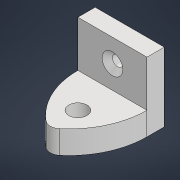
# Autodesk Inventor part: Winkel
Saved by Autodesk Inventor 2021 (Build 250183000, 183)
## iProperties
Created: 2023-10-25
Part Number: Winkel
Material: Generisch
Document SubType Name: Modeling
Designer: Tobias Sauter
Density: 1 g/cm^3
Appearance: Vorgabe
Author: Team 8
Autodesk Inventor part; units mm, degrees
ref_plane "YZ Plane" through (0, 0, 0) normal (1, 0, 0) x (0, 1, 0)
ref_plane "XZ Plane" through (0, 0, 0) normal (0, 1, 0) x (-1, 0, 0)
ref_plane "XY Plane" through (0, 0, 0) normal (0, 0, 1) x (1, 0, 0)
sketch "Skizze2" plane through (0, 0, 0) normal (0, 0, 1) x (1, 0, 0)
  line L0 (-36, 116.4167) -> (-56, 116.4167)
  line L1 (-56, 116.4167) -> (-56, 96.4167)
  line L2 (-56, 96.4167) -> (-36, 96.4167)
  line L3 (-36, 96.4167) -> (-36, 116.4167)
  circle A0 centre (-46, 109.75) radius 1.7 projected
  point P0 (0, 0)
  dimension "d0" = 20
  dimension "d1" = 10
  dimension "d2" = 20
  dimension "d3" = 6.6667
  constraints: 8 end point, 2 parallel, 1 horizontal, 1 perpendicular
  measures "d0" distance of L0.start L0.end
  measures "d1" distance from line of L3 A0.centre
  measures "d2" distance of L0.end L1.end
  measures "d3" distance from line of L0 A0.centre
extrude "Extrusion1" add sketch "Skizze2" along normal blind 5 contours L3 L2 L1 L0 | A0
sketch "Skizze4" plane through (-56, 96.4167, 0) normal (0, -1, 0) x (1, 0, 0)
  line L0 (0, 0) -> (20, 0) projected
  line L1 (20, 0) -> (20, 5) projected
  line L2 (0, 5) -> (20, 5) projected
  line L3 (0, 0) -> (0, 5) projected
  line L4 (0, 0) -> (0, 5) projected
  line L5 (20, 0) -> (20, 5) projected
  arc A0 (11.927, 22.2993) -> (8.073, 22.2993) centre (10, 20) ccw
  line L6 (10, 20) -> (10, 5) construction
  line L7 (0, 5) -> (20, 5) construction
  arc A1 (8.073, 22.2993) -> (0, 5) centre (22.5714, 5) ccw
  arc A2 (20, 5) -> (11.927, 22.2993) centre (-2.5714, 5) ccw
  circle A3 centre (10, 15) radius 2.65
  point P0 (56, 0)
  dimension "d6" = 6
  dimension "d7" = 15
  dimension "d8" = 23
  dimension "d11" = 5.3
  dimension "d20" = 10
  constraints: 6 point on circle, 4 centre point, 2 end point, 2 symmetric about line, 2 tangent, 1 midpoint, 1 perpendicular, 1 point on line, 1 other
  measures "d6" diameter of A0
  measures "d7" distance from line of L2 L6.start
  measures "d11" diameter of A3
  measures "d20" distance from line of L2 A3.centre
extrude "Extrusion2" add sketch "Skizze4" against normal blind 6.6667 contours A1 A0 A2 L2
sketch "Skizze6" plane through (0, 0, 5) normal (0, 0, 1) x (1, 0, 0)
  circle A0 centre (-46, 109.75) radius 1.7 projected
  point P0 (0, 0)
  constraints: 1 coincident
hole "Bohrung1" at (-46, 109.75, 5) direction (0, 0, -1) diameter 3 end through all countersink diameter 6 countersink angle 90
equation "\"d1\" = 0.5 * d0"
equation "\"d3\" = 0.333333 * d2"
